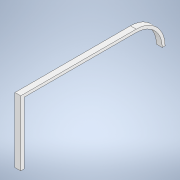
# Autodesk Inventor part: CONTAINER PIPE
Saved by Autodesk Inventor 2021 (Build 250183000, 183)
## iProperties
Created: 2021-07-10
Part Number: CONTAINER PIPE
Material: Generic
Document SubType Name: Modeling
Designer: HP
Density: 1 g/cm^3
Appearance: White
Author: HP
Autodesk Inventor part; units mm, degrees
ref_plane "YZ Plane" through (0, 0, 0) normal (1, 0, 0) x (0, 1, 0)
ref_plane "XZ Plane" through (0, 0, 0) normal (0, 1, 0) x (-1, 0, 0)
ref_plane "XY Plane" through (0, 0, 0) normal (0, 0, 1) x (1, 0, 0)
sketch "Sketch1" plane through (0, 0, 0) normal (1, 0, 0) x (0, 1, 0)
  line L0 (0, 10.0605) -> (0, 10.7499)
  arc A0 (0, -25.4) -> (25.4, 0) centre (0, 0) ccw
  arc A1 (0, -23.8125) -> (23.8125, 0) centre (0, 0) ccw
  line L1 (25.4, 0) -> (25.4, 101.6)
  line L2 (23.8125, 0) -> (23.8125, 101.6)
  line L3 (25.4, 101.6) -> (23.8125, 101.6)
  dimension "d2" = 25.4
  dimension "d3" = 101.6
  dimension "d4" = 101.6
  constraints: 8 end point, 4 point on circle, 2 centre point, 2 coincident, 2 vertical, 1 horizontal
  measures "d2" radius of A0
  measures "d3" distance of L1.start L1.end
  measures "d4" distance of L2.start L2.end
extrude "Extrusion1" [suppressed]
sketch "Sketch2" plane through (0, 0, 0) normal (1, 0, 0) x (0, 1, 0)
  arc A0 (0, -25.4) -> (25.4, 0) centre (0, 0) ccw
  arc A1 (0, -22.86) -> (22.86, 0) centre (0, 0) ccw
  line L0 (0, -22.86) -> (0, -25.4)
  line L1 (25.4, 0) -> (25.4, 101.6)
  line L2 (22.86, 0) -> (22.86, 98.425)
  line L3 (22.86, 98.425) -> (-6.35, 98.425)
  line L4 (-6.35, 98.425) -> (-6.35, 101.6)
  line L5 (-6.35, 101.6) -> (14.2875, 101.6)
  line L6 (14.2875, 101.6) -> (16.1645, 101.6)
  line L7 (16.1645, 101.6) -> (25.4, 101.6)
  dimension "d5" = 25.4
  dimension "d6" = 22.86
  dimension "d8" = 101.6
  constraints: 16 end point, 4 point on circle, 3 perpendicular, 3 vertical, 2 centre point, 2 coincident, 1 horizontal, 1 point on line
  measures "d5" radius of A0
  measures "d6" radius of A1
  measures "d8" distance of L1.start L1.end
extrude "Extrusion2" add sketch "Sketch2" along normal blind 5.08
sketch "Sketch3" plane through (0, -6.35, 98.425) normal (0, -1, 0) x (1, 0, 0)
  line L0 (5.08, -98.425) -> (5.08, 3.175) projected
  line L1 (0, 0) -> (5.08, 0) projected
  line L2 (5.08, 3.175) -> (0, 3.175)
  line L3 (0, 3.175) -> (0, 0)
  line L4 (0, 0) -> (5.08, 0)
  line L5 (5.08, 0) -> (5.08, 3.175)
  point P0 (0, -98.425)
  constraints: 8 end point, 2 parallel, 1 horizontal, 1 perpendicular
extrude "Extrusion3" add sketch "Sketch3" along normal blind 25.4
body "Solid1"
